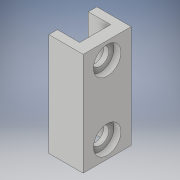
# Autodesk Inventor part: Schlitten_Part2
Saved by Autodesk Inventor 2019 (Build 230136000, 136)
## iProperties
Created: 2021-05-01
Part Number: Schlitten_Part2
Material: Generisch
Document SubType Name: Modeling
Designer: Bergi
Density: 1 g/cm^3
Appearance: Vorgabe
Author: Bergi
Autodesk Inventor part; units mm, degrees
ref_plane "YZ Plane" through (0, 0, 0) normal (1, 0, 0) x (0, 1, 0)
ref_plane "XZ Plane" through (0, 0, 0) normal (0, 1, 0) x (-1, 0, 0)
ref_plane "XY Plane" through (0, 0, 0) normal (0, 0, 1) x (1, 0, 0)
sketch "Skizze1" plane through (0, 0, 0) normal (0, 1, 0) x (-1, 0, 0)
  line L0 (-5, 7) -> (5, 7)
  line L1 (5, 7) -> (5, -7)
  line L2 (5, -7) -> (-5, -7)
  line L3 (-5, -7) -> (-5, 7)
  line L4 (-5, 7) -> (5, -7) construction
  line L5 (5, 7) -> (-5, -7) construction
  line L6 (5, 4.5) -> (-1.5, 4.5)
  line L7 (-1.5, 4.5) -> (-1.5, -4.5)
  line L8 (-1.5, -4.5) -> (5, -4.5)
  line L9 (5, -4.5) -> (5, 4.5)
  line L10 (5, 4.5) -> (-1.5, -4.5) construction
  line L11 (-1.5, 4.5) -> (5, -4.5) construction
  line L12 (7, 0) -> (-7, 0) projected
  point P0 (0, 0)
  point P1 (1.75, 0)
  point P2 (1.75, 0)
  dimension "d0" = 10
  dimension "d1" = 14
  dimension "d2" = 6.5
  dimension "d3" = 9
  constraints: 24 end point, 5 midpoint, 4 parallel, 2 horizontal, 2 perpendicular, 2 point on line
  measures "d0" distance of L1.end L2.end
  measures "d1" distance of L0.end L1.end
  measures "d2" distance of L8.end L7.end
  measures "d3" distance of L7.end L6.end
extrude "Extrusion1" add sketch "Skizze1" along normal blind 30 contours L0 L1 L6 L7 L12 L3 | L12 L7 L8 L1 L2 L3
sketch "Skizze2" plane through (5, 0, 7) normal (1, 0, 0) x (0, 0, -1)
  line L0 (7, -6) -> (7, 36) construction
  point P0 (7, 0)
  point P1 (7, 25)
  point P2 (7, 5)
  dimension "d6" = 20
  dimension "d7" = 5
  constraints: 2 point on line
  measures "d6" distance of point (7, 5) point (7, 25)
  measures "d7" distance of point (7, 0) point (7, 5)
hole "Bohrung1" at (5, 25, 0) at (5, 5, 0) direction (-1, 0, 0) diameter 5 end through all counterbore diameter 8 counterbore depth 2
